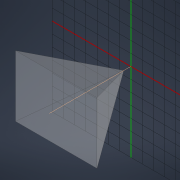
# Autodesk Inventor part: Camera-Viewcone
Saved by Autodesk Inventor 2022.2 (Build 262287010, 287A)
## iProperties
Created: 2022-04-02
Part Number: Camera-Viewcone
Material: Polycarbonat, klar
Document SubType Name: Modeling
Designer: sleib
Density: 1.2 g/cm^3
Appearance: Polycarbonat - klar
Author: sleib
Autodesk Inventor part; units mm, degrees
ref_plane "YZ Plane" through (0, 0, 0) normal (1, 0, 0) x (0, 1, 0)
ref_plane "XZ Plane" through (0, 0, 0) normal (0, 1, 0) x (-1, 0, 0)
ref_plane "XY Plane" through (0, 0, 0) normal (0, 0, 1) x (1, 0, 0)
sketch "Skizze1" plane through (0, 0, 0) normal (1, 0, 0) x (0, 1, 0)
  line L0 (0, 0) -> (272.1721, 600)
  line L1 (272.1721, 600) -> (-272.1721, 600)
  line L2 (-272.1721, 600) -> (0, 0)
  line L3 (0, 600) -> (0, 0) construction
  dimension "d0" = 48.8
  dimension "d1" = 600
  constraints: 8 end point, 1 horizontal, 1 midpoint, 1 vertical
  measures "d0" angle of L2 L0
  measures "d1" distance from line of L0.start L1
sketch "Skizze2" plane through (0, 0, 0) normal (0, 1, 0) x (-1, 0, 0)
  line L0 (0, 0) -> (361.9431, 600)
  line L1 (361.9431, 600) -> (-361.9431, 600)
  line L2 (-361.9431, 600) -> (0, 0)
  line L3 (0, 600) -> (0, 0) construction
  dimension "d2" = 62.2
  dimension "d3" = 600
  constraints: 8 end point, 1 horizontal, 1 midpoint, 1 vertical
  measures "d2" angle of L2 L0
  measures "d3" distance from line of L0.start L1
extrude "Extrusion1" add sketch "Skizze1" along normal mid plane 800
extrude "Extrusion2" cut sketch "Skizze2" along normal through all both and the other way through all keep common part
